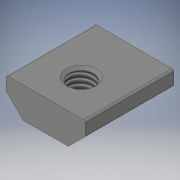
# Autodesk Inventor part: 40-1964
Saved by Autodesk Inventor 2019 (Build 230136000, 136)
## iProperties
Created: 2024-06-07
Part Number: 40-1964
Material: Generic
Catalog Web Link: www.cadenas.de
Description: 25-1954, 25-1964, 25-3204, 25-8901, 40-1964, 40-1984, 40-3202, 40-3203, 40-8900-Slide-In T-Nuts
Vendor: 8020
Document SubType Name: Modeling
Designer: psAdmin
Manufacturer: 8020
Mass: 1.41136 g
Surface Area: 9.26592 cm^2
Volume: 1.41136 cm^3
Density: 1 g/cm^3
Appearance: PSOLRGB-127-127-127
Category: PARTsolutions
Company: 8020
Title: 40-1964
Author: Cadenas PARTsolutions
Comments: Slide-In T-Nuts
PSOL_IDENT_0: {$CADENAS_DATA/23d-libs/8020/metric/fastening_options/25_1954.prj},228 {VTYP=3D},{NB=40-1964},{LINA=
PSOL_IDENT_1: 40-1964},{NN=25-1954, 25-1964, 25-3204, 25-8901, 40-1964, 40-1984, 40-3202, 40-3203, 40-8900},{DATE=
PSOL_IDENT_2: 16.06.2022 21:15:49},{GEOMDATE=15.05.2012 11:39:00},{VERSION=},{LINEID=180},{WBVAR=},{WBNUMERIC=}  {
PSOL_IDENT_3: NB=40-1964},{LINA=40-1964},{KT=DUMMY},{PN=40-1964},{MAT=1215 Carbon Steel},{FIN=Bright Zinc},{A=6.16
PSOL_IDENT_4: },{A1=6.15950},{B=7.14},{B1=7.13740},{C=17.78},{C1=17.78000},{D=15.88},{D1=15.87500},{E=M6 x 1.0},{E
PSOL_IDENT_5: 1=6.00000},{TT=M},{W=.0090},{COL=0.50,0.50,0.50,0.00},{NO=5}
NB: 40-1964
NN: 25-1954, 25-1964, 25-3204, 25-8901, 40-1964, 40-1984, 40-3202, 40-3203, 40-8900
NT: Slide-In T-Nuts
NBSYN: $PN.
LINA: 40-1964
CATALOG: 80/20
PN: 40-1964
MAT: 1215 Carbon Steel
FIN: Bright Zinc
A: 6.16
B: 7.14
C: 17.78
D: 15.88
E: M6 x 1.0
W: .0090
SUPPLIER: 8020
ARTICLENO: 40-1964
BOMINFO: 40-1964
CREATOR: CADENAS GmbH
Autodesk Inventor part; units mm, degrees
sketch "Sketch_1" plane through (0, 0, -10.6426) normal (0, 0, 1) x (1, 0, 0)
  line L0 (-7.9375, 5.7785) -> (-7.9375, 3.5455)
  arc A0 (-7.9375, 3.5455) -> (-7.8259, 3.2761) centre (-7.5565, 3.5455) ccw
  line L1 (-7.8259, 3.2761) -> (-4.6614, 0.1116)
  arc A1 (-4.6614, 0.1116) -> (-4.392, 0) centre (-4.392, 0.381) ccw
  line L2 (-4.392, 0) -> (4.392, 0)
  arc A2 (4.392, 0) -> (4.6614, 0.1116) centre (4.392, 0.381) ccw
  line L3 (4.6614, 0.1116) -> (7.8259, 3.2761)
  arc A3 (7.8259, 3.2761) -> (7.9375, 3.5455) centre (7.5565, 3.5455) ccw
  line L4 (7.9375, 3.5455) -> (7.9375, 5.7785)
  arc A4 (7.9375, 5.7785) -> (7.5565, 6.1595) centre (7.5565, 5.7785) ccw
  line L5 (7.5565, 6.1595) -> (-7.5565, 6.1595)
  arc A5 (-7.5565, 6.1595) -> (-7.9375, 5.7785) centre (-7.5565, 5.7785) ccw
  constraints: 12 end point, 12 point on circle, 6 centre point
extrude "Extrusion1" add sketch "Sketch_1" along normal blind 17.78
sketch "Sketch_4" plane through (0, 0, 0) normal (0, 0, 1) x (1, 0, 0)
  line L0 (0, 0) -> (0, 6.1595)
  line L1 (0, 6.1595) -> (3, 6.1595)
  line L2 (3, 6.1595) -> (2.4585, 5.618)
  line L3 (2.4585, 5.618) -> (2.4585, 0.5415)
  line L4 (2.4585, 0.5415) -> (3, 0)
  line L5 (3, 0) -> (0, 0)
  line L6 (0, 0) -> (0, 6.1595)
  constraints: 14 end point
revolve "Revolution1" cut sketch "Sketch_4" angle 360 about axis through (0, 0, 0) along (0, -1, 0)
thread "Thread1" size "M6x1" class "6H" standard "ISO Metric profile" full length
ref_plane "tnut_XY" through (0, 6.1595, 0) normal (0, 1, 0) x (1, 0, 0)
ref_plane "tnut_YZ" through (0, 6.1595, 0) normal (1, 0, 0) x (0, 0, -1)
ref_plane "tnut_ZX" through (0, 6.1595, 0) normal (0, 0, -1) x (0, 1, 0)
body "Solid1"
